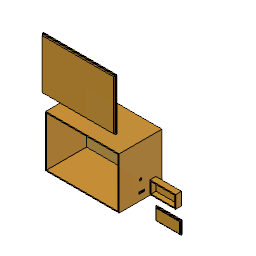
DISEÑO 3D taller de diseño (Autodesk Fusion 360 design; units mm, degrees)
part number: 2026-07-09-14-15-12-035
Autodesk Fusion 360 part; units mm, degrees
sketch "Boceto2" plane through (0, 0, 0) normal (0, 0, 1) x (1, 0, 0)
  line L0 (0, 0) -> (145, 0)
  line L1 (145, 0) -> (145, 100)
  line L2 (145, 100) -> (0, 100)
  line L3 (0, 100) -> (0, 0)
sketch "Boceto3" plane through (0, 0, 0) normal (0, 0, 1) x (1, 0, 0)
  line L0 (0, 0) -> (149, 0)
  line L1 (149, 0) -> (149, 104)
  line L2 (149, 104) -> (0, 104)
  line L3 (0, 104) -> (0, 0)
sketch "Boceto4" plane through (0, 0, 0) normal (0, 0, 1) x (1, 0, 0)
  line L0 (0, 0) -> (149, 0)
  line L1 (149, 0) -> (149, 104)
  line L2 (149, 104) -> (0, 104)
  line L3 (0, 104) -> (0, 0)
sketch "Boceto5" plane through (0, 0, 0) normal (0, 0, 1) x (1, 0, 0)
  line L0 (0, 0) -> (149, 0)
  line L1 (149, 0) -> (149, 104)
  line L2 (149, 104) -> (0, 104)
  line L3 (0, 104) -> (0, 0)
extrude "Extruir4" add sketch "Boceto5" along normal blind 87 makes body 1
ref_plane "PlanoDeObra1" through (0, 0, 87) normal (0, 0, 1) x (1, 0, 0)
sketch "Boceto6" plane through (0, 0, 87) normal (0, 0, 1) x (1, 0, 0)
  line L0 (2, 2) -> (147, 2)
  line L1 (147, 2) -> (147, 102)
  line L2 (147, 102) -> (2, 102)
  line L3 (2, 102) -> (2, 2)
extrude "Extruir5" cut sketch "Boceto6" against normal blind 85 bodies 1
sketch "Boceto7" plane through (0, 0, 0) normal (1, 0, 0) x (0, 0, -1)
sketch "Boceto8" plane through (0, 0, 2) normal (0, 0, 1) x (1, 0, 0)
  line L0 (2, 102) -> (2, 2)
  line L1 (2, 2) -> (147, 2)
  line L2 (147, 2) -> (147, 102)
  line L3 (147, 102) -> (2, 102)
  line L4 (2, 2) -> (147, 2)
  line L5 (147, 2) -> (147, 102)
  line L6 (147, 102) -> (2, 102)
  line L7 (2, 102) -> (2, 2)
  constraint horizontal L4
  constraint vertical L5
  constraint horizontal L6
  constraint vertical L7
  constraint coincident L2.end L3.start
  constraint coincident L0.end L1.start
extrude "Extruir6" add sketch "Boceto8" along normal blind 4 bodies 1
sketch "Boceto9" plane through (0, 0, 6) normal (0, 0, 1) x (1, 0, 0)
  line L0 (2, 102) -> (2, 2)
  line L1 (2, 2) -> (147, 2)
  line L2 (147, 2) -> (147, 102)
  line L3 (147, 102) -> (2, 102)
sketch "Boceto10" plane through (2, 0, 0) normal (1, 0, 0) x (0, 0, -1)
  line L0 (-6, 2) -> (-6, 102)
  line L1 (-6, 102) -> (-87, 102)
  line L2 (-87, 102) -> (-87, 2)
  line L3 (-87, 2) -> (-6, 2)
  line L4 (-46.8871, 16.5953) -> (-35.6071, 16.5953)
  line L5 (-35.6071, 16.5953) -> (-35.6071, 12.9253)
  line L6 (-35.6071, 12.9253) -> (-46.8871, 12.9253)
  line L7 (-46.8871, 12.9253) -> (-46.8871, 16.5953)
  circle A0 centre (-43.4879, 37.6172) radius 2.5
  dimension "d18" = 11.28
  dimension "d19" = 3.67
  dimension "d20" = 5
  constraint horizontal L4
  constraint vertical L5
  constraint horizontal L6
  constraint vertical L7
  measures "d18" distance of L4.start L4.end
  measures "d19" distance of L4.start L6.end
  measures "d20" diameter of A0
ref_plane "PlanoDeObra2" through (0, 0, 87) normal (0, 0, 1) x (1, 0, 0)
sketch "Boceto11" plane through (0, 0, 87) normal (0, 0, 1) x (1, 0, 0)
  line L0 (0, 0) -> (149, 0)
  line L1 (149, 0) -> (149, 104)
  line L2 (149, 104) -> (0, 104)
  line L3 (0, 104) -> (0, 0)
extrude "Extruir7" add sketch "Boceto11" along normal blind 2 separate body makes body 2
move_body "Desplazar1" bodies 2 to x (1, 0, 0) y (0, 1, 0) z (0, 0, 1) at (0, 0, 40)
ref_plane "PlanoDeObra3" through (0, 0, 127) normal (0, 0, 1) x (1, 0, 0)
sketch "Boceto12" plane through (0, 0, 127) normal (0, 0, 1) x (1, 0, 0)
  line L0 (2, 2) -> (147, 2)
  line L1 (147, 2) -> (147, 102)
  line L2 (147, 102) -> (2, 102)
  line L3 (2, 102) -> (2, 2)
  line L4 (4, 4) -> (145, 4)
  line L5 (145, 4) -> (145, 100)
  line L6 (145, 100) -> (4, 100)
  line L7 (4, 100) -> (4, 4)
extrude "Extruir8" add sketch "Boceto12" against normal blind 3 bodies 2
extrude "Extruir9" add 1 faces at (51, 68, 127) along direction (0, 0, -1) blind 2 on bodies 2 bodies 2
extrude "Extruir10" add 1 faces at (51, 68, 125) along direction (0, 0, -1) blind 1 on bodies 2 bodies 2
sketch "Boceto13" plane through (0, 0, 0) normal (0, 0, 1) x (1, 0, 0)
  line L0 (0, 160) -> (52, 160)
  line L1 (52, 160) -> (52, 186)
  line L2 (52, 186) -> (0, 186)
  line L3 (0, 186) -> (0, 160)
extrude "Extruir11" add sketch "Boceto13" along normal blind 12 separate body makes body 3
sketch "Boceto14" plane through (0, 0, 0) normal (0, 0, 1) x (1, 0, 0)
  line L0 (2, 162) -> (50, 162)
  line L1 (50, 162) -> (50, 184)
  line L2 (50, 184) -> (2, 184)
  line L3 (2, 184) -> (2, 162)
extrude "Extruir12" add sketch "Boceto14" along normal blind 10.01 separate body makes body 4
combine "Combinar1" operation cut target body 3 tool bodies 4
sketch "Boceto15" plane through (0, 0, 0) normal (0, 0, 1) x (1, 0, 0)
  line L0 (0, 191) -> (52, 191)
  line L1 (52, 191) -> (52, 217)
  line L2 (52, 217) -> (0, 217)
  line L3 (0, 217) -> (0, 191)
extrude "Extruir13" add sketch "Boceto15" along normal blind 2 separate body makes body 5
sketch "Boceto16" plane through (0, 0, 0) normal (0, 0, 1) x (1, 0, 0)
  line L0 (2.1, 193.1) -> (49.9, 193.1)
  line L1 (49.9, 193.1) -> (49.9, 214.9)
  line L2 (49.9, 214.9) -> (2.1, 214.9)
  line L3 (2.1, 214.9) -> (2.1, 193.1)
extrude "Extruir14" add sketch "Boceto16" along normal mid plane 3 bodies 5
move_body "Desplazar2" bodies 3 to x (1, 0, 0) y (0, -1, 0) z (0, 0, -1) at (0, 268.2898, 80.5073)
move_body "Desplazar3" bodies 3 to x (1, 0, 0) y (0, 1, 0) z (0, 0, 1) at (0, 150, 0)
move_body "Desplazar4" bodies 5 to x (1, 0, 0) y (0, 1, 0) z (0, 0, 1) at (75, 0, 0)
move_body "Desplazar5" bodies 2 to x (1, 0, 0) y (0, 1, 0) z (0, 0, 1) at (0, 55.7743, 37.2012)
move_body "Desplazar6" bodies 2 5 to x (1, 0, 0) y (0, 1, 0) z (0, 0, 1) at (175, -50, 0)
move_body "Desplazar7" bodies 3 to x (1, 0, 0) y (0, 1, 0) z (0, 0, 1) at (575, -175, 0)
move_body "Desplazar8" bodies 5 to x (1, 0, 0) y (0, -1, 0) z (0, 0, -1) at (100, 308, 4)
move_body "Desplazar9" bodies 2 to x (1, 0, 0) y (0, -1, 0) z (0, 0, -1) at (0, 115.5486, 332.4023)
move_body "Desplazar10" bodies 3 to x (1, 0, 0) y (0, 1, 0) z (0, 0, 1) at (-200, 0, 0)
move_body "Desplazar11" bodies 2 to x (1, 0, 0) y (0, 1, 0) z (0, 0, 1) at (-190, 120, 0)
move_body "Desplazar12" bodies 5 to x (1, 0, 0) y (0, 1, 0) z (0, 0, 1) at (-140, -130, 0)
move_body "Desplazar13" bodies 3 to x (1, 0, 0) y (0, 1, 0) z (0, 0, 1) at (-170, 0, 0)
move_body "Desplazar14" bodies 5 to x (1, 0, 0) y (0, 1, 0) z (0, 0, 1) at (0, 0, 70)
move_body "Desplazar15" bodies 2 to x (1, 0, 0) y (0, 1, 0) z (0, 0, 1) at (0, 0, -90)
extrude "Extruir15" cut sketch "Boceto10" along normal through all contours A0 bodies 1
extrude "Extruir16" cut sketch "Boceto10" along normal through all contours L4 L5 L6 L7 bodies 1
named bodies: "Caja interior 145x100x85mm", "Tapa 149x104x2mm", "Caja_48x22x10", "CUT_interior", "Tapa_48x22"
